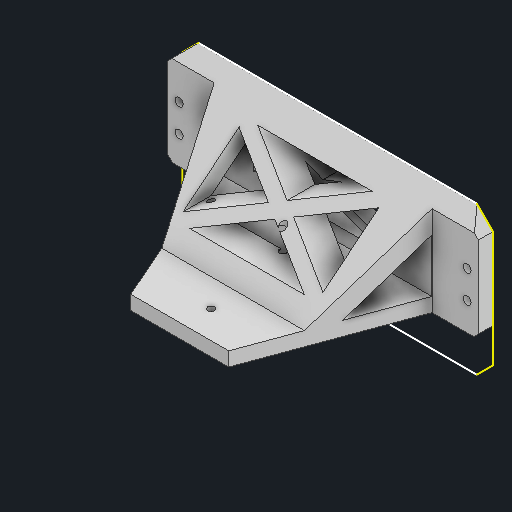
# Autodesk Inventor part: Stepper_holder
Saved by Autodesk Inventor 2026.1 (Build 301233020, 233B)
## iProperties
Created: 2026-03-04
Part Number: Stepper_holder
Material: Generic
Document SubType Name: Modeling
Designer: Mikke
Density: 1 g/cm^3
Appearance: Default
Author: Mikke
Autodesk Inventor part; units mm, degrees
ref_plane "YZ Plane" through (0, 0, 0) normal (1, 0, 0) x (0, 1, 0)
ref_plane "XZ Plane" through (0, 0, 0) normal (0, 1, 0) x (-1, 0, 0)
ref_plane "XY Plane" through (0, 0, 0) normal (0, 0, 1) x (1, 0, 0)
sketch "Sketch1" plane through (0, 0, 0) normal (0, 0, 1) x (1, 0, 0)
  line L0 (6.4, -25) -> (-0.5799, -31.9799) projected
  line L1 (6.4, 25) -> (6.4, -25) projected
  line L2 (-0.5799, 31.9799) -> (6.4, 25) projected
  line L3 (-120.6201, 31.9799) -> (-127.6, 25) projected
  line L4 (-127.6, 25) -> (-127.6, -25) projected
  line L5 (-127.6, -25) -> (-120.6201, -31.9799) projected
  circle A0 centre (1.5276, -12) radius 1.75 projected
  circle A1 centre (1.5276, 0) radius 1.75 projected
  circle A2 centre (1.5276, 12) radius 1.75 projected
  circle A3 centre (-122.7276, 12) radius 1.75 projected
  circle A4 centre (-122.7276, 0) radius 1.75 projected
  circle A5 centre (-122.7276, -12) radius 1.75 projected
  line L6 (-0.5799, -31.9799) -> (-120.6201, -31.9799)
  line L7 (-120.6201, 31.9799) -> (-0.5799, 31.9799)
  point P0 (0, 0)
  constraints: 4 end point, 1 horizontal, 1 parallel
sketch "Sketch2" plane through (0, 0, 0) normal (1, 0, 0) x (0, 1, 0)
  line L0 (-132.1, 60.2267) -> (-132.1, 25.9267) projected
  line L1 (-132.1, 60.2267) -> (-102.6604, 60.2267) construction
  line L2 (-132.1, 25.9267) -> (-125.3433, 25.9267) construction
  line L3 (-6.0833, 46.5895) -> (31.7742, 0.0646)
  line L4 (31.7742, 0.0646) -> (-12.1352, 0)
  line L5 (-6.0833, 6.3314) -> (-6.0833, 34.528)
  line L6 (-6.0833, 34.528) -> (16.9694, 6.3314)
  line L7 (16.9694, 6.3314) -> (-6.0833, 6.3314)
  line L8 (-12.1352, 0) -> (-12.1352, 70.4961)
  line L9 (-12.1352, 0) -> (31.7742, 0.0646)
  line L10 (-6.0833, 46.5895) -> (-6.0833, 70.4961)
  line L11 (-6.0833, 70.4961) -> (-12.1352, 70.4961)
  point P0 (0, 0)
  constraints: 22 end point, 3 vertical, 2 horizontal, 2 perpendicular, 1 collinear
extrude "Extrusion1" add sketch "Sketch2" against normal blind 127.6
sketch "Sketch4" plane through (0, 0, 0) normal (1, 0, 0) x (0, 0, -1)
  line L0 (-0.0646, 31.7742) -> (-46.5895, -6.0833) projected
  line L1 (-70.4961, -12.1352) -> (0, -12.1352) projected
  line L2 (0, -12.1352) -> (-0.0646, 31.7742) projected
  line L3 (-6.3314, -6.0833) -> (-34.528, -6.0833) projected
  line L4 (-34.528, -6.0833) -> (-6.3314, 16.9694) projected
  line L5 (-6.3314, 16.9694) -> (-6.3314, -6.0833) projected
  line L6 (-46.5895, -6.0833) -> (-70.4961, -6.0833) projected
  line L7 (-70.4961, -6.0833) -> (-70.4961, -12.1352) projected
  point P0 (0, 0)
extrude "Extrusion3" add sketch "Sketch4" along normal blind 6.4
sketch "Sketch6" plane through (-127.6, -12.1352, 0) normal (0, -1, 0) x (1, 0, 0)
  line L0 (134, 70.4962) -> (0, 70.4962) projected
  line L1 (0, 0) -> (0, 70.4962) projected
  line L2 (0, 0) -> (134, 0) projected
  line L3 (134, 70.4962) -> (134, 0) projected
  line L4 (134, 0) -> (134, 6.289)
  line L5 (134, 6.289) -> (114, 6.289)
  line L6 (0, 0) -> (0, 6.289)
  line L7 (0, 0) -> (0, 70.4962) projected
  line L8 (0, 6.289) -> (20, 6.289)
  line L9 (76.6176, 60.2267) -> (76.6176, 25.9267) projected
  line L10 (34.3176, 25.9267) -> (34.3176, 60.2267) projected
  line L11 (114, 6.289) -> (90.487, 70.4962)
  line L12 (20, 6.289) -> (48.187, 70.4962)
  line L13 (134, 70.4962) -> (0, 70.4962) projected
  point P0 (127.6, 0)
  dimension "d9" = 6.289
  dimension "d10" = 20
  dimension "d11" = 6.289
  dimension "d12" = 20
  constraints: 12 end point, 4 point on line, 2 perpendicular
  measures "d9" distance of L2.end L4.end
  measures "d10" distance of L4.end L5.end
  measures "d11" distance of L1.start L6.end
  measures "d12" distance of L6.end L8.end
extrude "Extrusion4" cut sketch "Sketch6" against normal blind 57.2 contours L3 L5 L11 L0 | L12 L8 L1 L0
sketch "Sketch7" plane through (6.4, -12.1352, 0) normal (0, 0.0014716, -0.9999989) x (-1, 0, 0)
  line L0 (6.9799, 44.115) -> (0, 37.1351) projected
  line L1 (127.0201, 44.115) -> (134, 37.1351) projected
  line L2 (134, 43.9094) -> (134, 0) projected
  line L3 (134, 37.1351) -> (134, 43.9094)
  line L4 (134, 43.9094) -> (127.0201, 44.115)
  line L5 (0, 0) -> (0, 43.9094) projected
  line L6 (0, 37.1351) -> (0, 43.9094)
  line L7 (0, 43.9094) -> (6.9799, 44.115)
  ellipse E0 centre (129.1276, 24.129) end of major axis (127.3776, 24.129) minor radius 1.75 projected
  ellipse E1 centre (129.1276, 12.129) end of major axis (127.3776, 12.129) minor radius 1.75 projected
  ellipse E2 centre (4.8724, 12.129) end of major axis (6.6224, 12.129) minor radius 1.75 projected
  ellipse E3 centre (4.8724, 24.129) end of major axis (6.6224, 24.129) minor radius 1.75 projected
  line L8 (134, 0) -> (0, 0) projected
  line L9 (134, 43.9094) -> (134, 0) projected
  line L10 (134, 43.9094) -> (0, 43.9094) projected
  line L11 (0, 0) -> (0, 43.9094) projected
  line L12 (20.0155, 6.0612) -> (113.9814, 6.0612) projected
  line L13 (121.5903, 6.0612) -> (15.751, 6.0612)
  line L14 (15.751, 6.0612) -> (15.751, 36.0612)
  line L15 (20, 0.0093) -> (20, 38.8538) projected
  line L16 (15.751, 6.0612) -> (45.751, 6.0612) construction
  line L17 (15.751, 36.0612) -> (41.7318, 21.0612)
  line L18 (41.7318, 21.0612) -> (15.751, 6.0612)
  line L19 (121.5903, 6.0612) -> (121.5903, 36.0612)
  line L20 (121.5903, 6.0612) -> (151.5903, 6.0612) construction
  line L21 (121.5903, 36.0612) -> (95.6095, 21.0612)
  line L22 (95.6095, 21.0612) -> (121.5903, 6.0612)
  point P0 (6.4, 12.1352)
  dimension "d20" = 30
  dimension "d21" = 90
  dimension "d22" = 30
  dimension "d23" = 30
  dimension "d24" = 30
  dimension "d25" = 90
  dimension "d26" = 30
  constraints: 26 end point, 2 collinear, 2 horizontal, 2 perpendicular, 1 parallel, 1 point on line, 1 vertical, 2 other
  measures "d20" distance of L13.end L14.end
  measures "d21" angle of L16 L14
  measures "d22" distance of L14.end L17.end
  measures "d23" distance of L17.end L13.end
  measures "d24" distance of L13.start L19.end
  measures "d25" angle of L20 L19
  measures "d26" distance of L19.end L21.end
extrude "Extrusion5" cut sketch "Sketch7" against normal blind 57.2 contours L0 L10 L7 | L0 L5 L10 | L10 L2 L1 | L1 L4 L10 | E0 | E1 | E2 | E3
chamfer "Chamfer1" distance 2 angle 45 2 edges at (6.4, -12.1352, 3.1445) (-127.6, -12.1352, 3.1445)
sketch "Sketch8" plane through (-0.3743, 31.7742, 0.0646) normal (0, 0.0014716, -0.9999989) x (-1, 0, 0)
  line L0 (90.3674, -7.9133) -> (30.0427, -7.9133)
  line L1 (30.0427, -7.9133) -> (30.0427, -31.7743)
  line L2 (30.0427, -31.7743) -> (90.3674, -31.7743)
  line L3 (90.3674, -31.7743) -> (90.3674, -7.9133)
  line L4 (90.3674, -7.9133) -> (30.0427, -31.7743) construction
  line L5 (30.0427, -7.9133) -> (90.3674, -31.7743) construction
  line L6 (90.3674, -31.7743) -> (30.0427, -7.9133)
  line L7 (30.0427, -31.7743) -> (90.3674, -7.9133)
  line L8 (29.3071, -9.7731) -> (89.6318, -33.6341)
  line L9 (30.7784, -6.0535) -> (91.1031, -29.9145)
  line L10 (91.1031, -9.7731) -> (30.7784, -33.6341)
  line L11 (89.6318, -6.0535) -> (29.3071, -29.9145)
  point P0 (-0.3743, -31.7743)
  point P1 (60.2051, -19.8438)
  point P2 (60.2051, -17.693)
  point P3 (84.9299, -7.9133)
  point P4 (35.4803, -7.9133)
  point P5 (30.0427, -29.6235)
  point P6 (54.7676, -19.8438)
  point P7 (30.0427, -10.0641)
  point P8 (60.2051, -21.9946)
  point P9 (35.4803, -31.7743)
  point P10 (84.9299, -31.7743)
  point P11 (90.3674, -10.0641)
  point P12 (65.6426, -19.8438)
  point P13 (90.3674, -29.6235)
  dimension "d27" = 2
  dimension "d28" = 2
  dimension "d29" = 2
  dimension "d30" = 2
  constraints: 24 end point, 7 equal length, 2 midpoint, 1 horizontal, 1 perpendicular
  measures "d27" distance between parallel lines of L5 L8
  measures "d28" distance between parallel lines of L5 L9
  measures "d29" distance between parallel lines of L4 L10
  measures "d30" distance between parallel lines of L4 L11
extrude "Extrusion6" cut sketch "Sketch8" against normal blind 57.2 contours L11 L9 L0 | L3 L9 L10 | L8 L11 L1 | L2 L10 L8
sketch "Sketch9" plane through (-79.413, -12.1352, 70.4961) normal (0, -1, 0) x (1, 0, 0)
  circle A0 centre (22.7806, -11.9195) radius 1.5 projected
  circle A1 centre (-8.2194, -11.9195) radius 1.5 projected
  circle A2 centre (-8.2194, -42.9195) radius 1.5 projected
  circle A3 centre (22.7806, -42.9195) radius 1.5 projected
  point P0 (79.413, -70.4961)
extrude "Extrusion7" cut sketch "Sketch9" against normal blind 34.975
sketch "Sketch10" plane through (-107.5814, -6.0833, 6.3314) normal (0, 1, 0) x (1, 0, 0)
  circle A0 centre (32.2202, -97.8435) radius 5
  circle A1 centre (1.2202, -97.8435) radius 5
  circle A2 centre (19.949, -52.2453) radius 1.5 projected
  circle A3 centre (50.949, -52.2453) radius 1.5 projected
  point P0 (107.5814, 6.3314)
  dimension "d35" = 10
  dimension "d36" = 10
  constraints: 2 centre point
  measures "d35" diameter of A0
  measures "d36" diameter of A1
extrude "Extrusion8" cut sketch "Sketch10" along normal blind 34.975 contours A0 | A1
body "Solid1"
